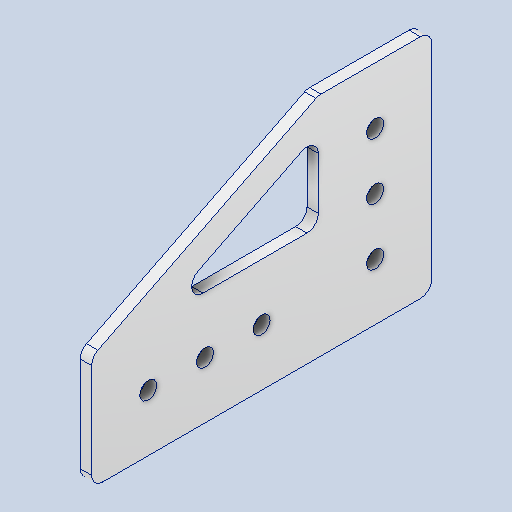
# Autodesk Inventor part: dribl-v1-Plate-9
Saved by Autodesk Inventor 2025.2 (Build 292293000, 293)
## iProperties
Created: 2025-01-13
Part Number: dribl-v1-Plate-9
Material: アルミニウム 6061
Document SubType Name: Modeling
Designer: haruy
Density: 2.7 g/cm^3
Appearance: アルミニウム - フラット
Author: haruy
Autodesk Inventor part; units mm, degrees
ref_plane "YZ Plane" through (0, 0, 0) normal (1, 0, 0) x (0, 1, 0)
ref_plane "XZ Plane" through (0, 0, 0) normal (0, 1, 0) x (-1, 0, 0)
ref_plane "XY Plane" through (0, 0, 0) normal (0, 0, 1) x (1, 0, 0)
sketch "スケッチ1" plane through (0, 0, 0) normal (1, 0, 0) x (0, 1, 0)
  line L0 (-65.3332, -639.5232) -> (-65.3332, 668.4768)
  line L1 (-65.3332, -537.5232) -> (339.6668, -537.5232)
  line L2 (339.6668, -537.5232) -> (339.6668, -517.5232)
  line L3 (339.6668, -517.5232) -> (-65.3332, -517.5232)
  line L4 (-65.3332, -517.5232) -> (-65.3332, -537.5232)
  circle A0 centre (-30.1532, -490.5232) radius 21
  circle A1 centre (-30.1532, -448.5232) radius 16
  circle A2 centre (-30.1532, -448.5232) radius 13.68
  line L5 (-85.3332, -639.5232) -> (-65.3332, -639.5232)
  line L6 (-85.3332, -639.5232) -> (-65.3332, -639.5232)
  line L7 (-85.3332, -639.5232) -> (398.6668, -639.5232)
  line L8 (398.6668, -639.5232) -> (398.6668, -659.5232)
  line L9 (398.6668, -659.5232) -> (-85.3332, -659.5232)
  line L10 (-85.3332, -659.5232) -> (-85.3332, -639.5232)
  line L11 (-10.1532, 668.4768) -> (9.0226, 674.1594)
  line L12 (9.0226, 674.1594) -> (394.8699, -627.872)
  line L13 (394.8699, -627.872) -> (375.6942, -633.5546)
  line L14 (375.6942, -633.5546) -> (-10.1532, 668.4768)
  line L15 (-85.3332, 668.4768) -> (-85.3332, -639.5232)
  line L16 (-85.3332, -432.5232) -> (-30.1532, -432.5232)
  line L17 (-9.1532, -490.5232) -> (-9.1532, -537.5232)
  line L18 (-9.1532, -490.5232) -> (-9.1532, -432.5232)
  line L19 (-9.1532, -432.5232) -> (-30.1532, -432.5232)
  circle A3 centre (-75.3332, -444.5232) radius 1.5
  circle A4 centre (-75.3332, -454.5232) radius 1.5
  line L20 (-30.1532, -464.5232) -> (-85.3332, -464.5232)
  circle A5 centre (-55.3332, -527.5232) radius 1.5
  circle A6 centre (-35.3332, -527.5232) radius 1.5
  line L21 (-65.3332, -537.5232) -> (-85.3332, -537.5232)
  circle A7 centre (-75.3332, -527.5232) radius 1.5
  circle A8 centre (-75.3332, -507.5232) radius 1.5
  circle A9 centre (-30.1532, 652.4768) radius 16
  line L22 (-65.3332, 668.4768) -> (-85.3332, 668.4768)
  line L23 (-85.3332, 668.4768) -> (-30.1532, 668.4768)
  line L24 (-30.1532, 636.4768) -> (-85.3332, 636.4768)
  line L25 (-30.1532, 668.4768) -> (-10.1532, 668.4768)
  circle A10 centre (-30.1532, 652.4768) radius 7.5
  line L26 (-30.1532, 636.4768) -> (-0.6702, 636.4768)
  circle A11 centre (-75.3332, 656.4768) radius 1.5
  circle A12 centre (-75.3332, 646.4768) radius 1.5
  circle A13 centre (2.276, 661.7302) radius 1.5
  circle A14 centre (5.1173, 652.1424) radius 1.5
  line L27 (-0.6702, 636.4768) -> (18.5055, 642.1594)
  line L28 (-65.3332, -599.5232) -> (-45.3332, -639.5232)
  line L29 (-45.3332, -639.5232) -> (-45.3332, -659.5232)
  line L30 (-65.3332, -599.5232) -> (-85.3332, -599.5232)
  circle A15 centre (-75.3332, -629.5232) radius 1.5
  circle A16 centre (-75.3332, -619.5232) radius 1.5
  circle A17 centre (-75.3332, -609.5232) radius 1.5
  circle A18 centre (-75.3332, -649.5232) radius 1.5
  circle A19 centre (-65.3332, -649.5232) radius 1.5
  circle A20 centre (-55.3332, -649.5232) radius 1.5
  line L31 (-85.3332, -639.5232) -> (-85.3332, -599.5232)
  line L32 (368.6668, -639.5232) -> (368.6668, -659.5232)
  line L33 (367.1703, -604.7911) -> (386.346, -599.1085)
  line L34 (375.6942, -633.5546) -> (377.4629, -639.5232)
  line L35 (394.8699, -627.872) -> (398.6668, -639.5232)
  circle A21 centre (378.6668, -649.5232) radius 1.5
  circle A22 centre (388.6668, -649.5232) radius 1.5
  circle A23 centre (382.4407, -621.1255) radius 1.5
  circle A24 centre (379.5994, -611.5376) radius 1.5
  circle A25 centre (319.6668, -527.5232) radius 1.5
  circle A26 centre (329.6668, -527.5232) radius 1.5
  line L36 (339.6668, -517.5232) -> (341.3091, -517.5232)
  line L37 (339.6668, -537.5232) -> (347.236, -537.5232)
  line L38 (341.3091, -517.5232) -> (362.1688, -517.5232)
  circle A27 centre (354.5961, -527.1644) radius 1.5
  circle A28 centre (357.4374, -536.7523) radius 1.5
  line L39 (350.6908, -549.1815) -> (369.8665, -543.4989)
  line L40 (309.6668, -517.5232) -> (309.6668, -537.5232)
  line L41 (-50.3332, -659.5232) -> (-50.3332, -640.7035)
  line L42 (-50.3332, -640.7035) -> (-68.4233, -604.5232)
  line L43 (-68.4233, -604.5232) -> (-80.3332, -604.5232)
  line L44 (-80.3332, -604.5232) -> (-80.3332, -639.5232)
  point P0 (0, 0)
  point P1 (-388.3332, -207.1898)
  point P2 (-65.3332, -517.5232)
  point P3 (385.282, -630.7133)
  point P4 (-50.9233, -639.5232)
  point P5 (-65.3332, -610.7035)
  dimension "d1" = 42
  dimension "d0" = 20
  dimension "d2" = 32
  dimension "d3" = 27.36
  dimension "d4" = 35.18
  dimension "d5" = 35.18
  dimension "d6" = 27
  dimension "d7" = 42
  dimension "d8" = 191
  dimension "d9" = 20
  dimension "d10" = 484
  dimension "d11" = 3
  dimension "d12" = 3
  dimension "d13" = 10
  dimension "d14" = 10
  dimension "d15" = 10
  dimension "d16" = 10
  dimension "d17" = 3
  dimension "d18" = 3
  dimension "d19" = 10
  dimension "d20" = 20
  dimension "d21" = 10
  dimension "d22" = 10
  dimension "d23" = 3
  dimension "d24" = 3
  dimension "d25" = 10
  dimension "d26" = 20
  dimension "d27" = 10
  dimension "d28" = 10
  dimension "d29" = 20
  dimension "d30" = 32
  dimension "d31" = 35.18
  dimension "d32" = 20
  dimension "d33" = 1358
  dimension "d34" = 91.543
  dimension "d35" = 405
  dimension "d36" = 15
  dimension "d37" = 3
  dimension "d38" = 3
  dimension "d39" = 10
  dimension "d40" = 10
  dimension "d41" = 10
  dimension "d42" = 10
  dimension "d43" = 3
  dimension "d44" = 3
  dimension "d45" = 10
  dimension "d46" = 10
  dimension "d47" = 10
  dimension "d48" = 10
  dimension "d49" = 40
  dimension "d50" = 3
  dimension "d51" = 3
  dimension "d52" = 3
  dimension "d53" = 3
  dimension "d54" = 3
  dimension "d55" = 3
  dimension "d56" = 10
  dimension "d57" = 10
  dimension "d58" = 10
  dimension "d59" = 10
  dimension "d60" = 10
  dimension "d61" = 10
  dimension "d62" = 10
  dimension "d63" = 10
  dimension "d64" = 10
  constraints: 90 end point, 28 centre point, 28 point on line, 14 perpendicular, 7 parallel, 7 tangent, 5 point on circle, 3 horizontal, 3 vertical, 2 coincident, 2 collinear, 1 horizontal alignment, 1 midpoint, 5 other
  measures "d0" distance of L2.end L1.end
  measures "d2" diameter of A1
  measures "d3" diameter of A2
  measures "d4" distance from line of L0 A1.centre
  measures "d5" distance from line of point (-30.153, -490.523) L0
  measures "d6" distance from line of L3 point (-30.153, -490.523)
  measures "d7" distance of point (-30.153, -490.523) A1.centre
  measures "d8" distance from line of A1.centre L5
  measures "d9" distance of L7.end L8.end
  measures "d10" distance between parallel lines of L10 L8
  measures "d11" diameter of A3
  measures "d12" diameter of A4
  measures "d13" distance of A4.centre A3.centre
  measures "d14" distance from line of A3.centre L0
  measures "d15" distance from line of A4.centre L20
  measures "d16" distance from line of L0 A4.centre
  measures "d17" diameter of A5
  measures "d18" diameter of A6
  measures "d19" distance from line of A5.centre L0
  measures "d20" distance of A6.centre A5.centre
  measures "d21" distance from line of A5.centre L1
  measures "d22" distance from line of A6.centre L1
  measures "d23" diameter of A7
  measures "d24" diameter of A8
  measures "d25" distance from line of A7.centre L21
  measures "d26" distance of A8.centre A7.centre
  measures "d27" distance from line of A8.centre L15
  measures "d28" distance from line of L15 A7.centre
  measures "d29" distance between parallel lines of L14 L12
  measures "d30" diameter of A9
  measures "d31" distance from line of L0 A9.centre
  measures "d32" horizontal distance of L11.start A9.centre
  measures "d33" distance between parallel lines of L11 L13
  measures "d35" distance between parallel lines of L0 L2
  measures "d36" diameter of A10
  measures "d37" diameter of A11
  measures "d38" diameter of A12
  measures "d39" distance from line of A12.centre L24
  measures "d40" distance of A11.centre A12.centre
  measures "d41" distance from line of A12.centre L0
  measures "d42" distance from line of A11.centre L0
  measures "d43" diameter of A13
  measures "d44" diameter of A14
  measures "d45" distance from line of A13.centre L11
  measures "d46" distance from line of A13.centre L12
  measures "d47" distance of A13.centre A14.centre
  measures "d48" distance from line of A14.centre L12
  measures "d49" distance between parallel lines of L10 L29
  measures "d50" diameter of A15
  measures "d51" diameter of A16
  measures "d52" diameter of A17
  measures "d53" diameter of A18
  measures "d54" diameter of A19
  measures "d55" diameter of A20
  measures "d56" distance from line of A18.centre L9
  measures "d57" distance from line of A18.centre L10
  measures "d58" distance of A19.centre A18.centre
  measures "d59" distance from line of A19.centre L9
  measures "d60" distance from line of A20.centre L9
  measures "d61" distance of A19.centre A20.centre
  measures "d62" distance from line of A15.centre L7
  measures "d63" distance from line of A15.centre L0
  measures "d64" distance of A16.centre A15.centre
extrude "押し出し1" add sketch "スケッチ1" against normal blind 2 contours L28 L7 L42 L0 | L0 L42 L43 L44 L5 L15 L30 | L42 L7 L0 | L0 L5 L44 L43 L42 | L29 L9 L41 L42 L7 | L7 L42 L41 L9 L10 L5
extrude "押し出し2" cut sketch "スケッチ1" against normal blind 2 contours L42 L7 L0
fillet "フィレット1" radius 2 8 edges at (-1, -85.3332, -599.5232) (-1, -65.3332, -599.5232) (-1, -65.3332, -610.7035) (-1, -65.3332, -639.5232) (-1, -50.9233, -639.5232) (-1, -45.3332, -639.5232) (-1, -45.3332, -659.5232) (-1, -85.3332, -659.5232)
equation "\"d5\" = d4"
equation "\"d14\" = d15"
equation "\"d21\" = d19"
equation "\"d22\" = d19"
equation "\"d27\" = d25"
equation "\"d28\" = d25"
equation "\"d31\" = d4"
equation "\"d41\" = d39"
equation "\"d42\" = d39"
equation "\"d46\" = d45"
equation "\"d47\" = d45"
equation "\"d48\" = d45"
equation "\"d57\" = d56"
equation "\"d58\" = d56"
equation "\"d59\" = d56"
equation "\"d60\" = d56"
equation "\"d61\" = d56"
equation "\"d62\" = d56"
equation "\"d63\" = d56"
equation "\"d64\" = d62"
